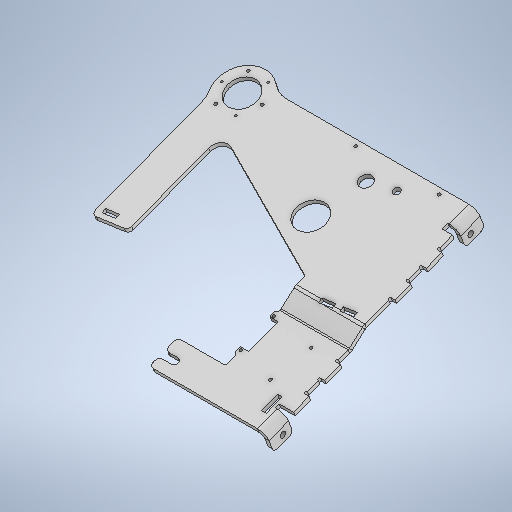
# Autodesk Inventor part: 21-30-220-B1
Saved by Autodesk Inventor 2025.2 (Build 292293000, 293)
## iProperties
Created: 2024-12-03
Part Number: 21-30-220-B1
Material: Generic
Document SubType Name: Sheet Metal
Designer: Zvonko.Gabric
Density: 1 g/cm^3
Sheet Metal Rule: Default_mm
Appearance: Default
Author: Zvonko.Gabric
Autodesk Inventor part; units mm, degrees
ref_plane "YZ Plane" through (0, 0, 0) normal (1, 0, 0) x (0, 1, 0)
ref_plane "XZ Plane" through (0, 0, 0) normal (0, 1, 0) x (-1, 0, 0)
ref_plane "XY Plane" through (0, 0, 0) normal (0, 0, 1) x (1, 0, 0)
sketch "Sketch1" plane through (0, 0, 0) normal (0, 1, 0) x (-1, 0, 0)
  line L0 (0, 0) -> (135, 0)
  line L1 (140, -5) -> (140, -6.9)
  line L2 (135, -11.9) -> (124, -11.9)
  line L3 (124, -11.9) -> (124, -20.1) construction
  line L4 (124, -20.1) -> (135, -20.1)
  line L5 (140, -25.1) -> (140, -31)
  line L6 (135, -36) -> (85, -36)
  arc A0 (124, -11.9) -> (124, -20.1) centre (124, -16) ccw
  arc A1 (140, -5) -> (135, 0) centre (135, -5) ccw
  arc A2 (135, -11.9) -> (140, -6.9) centre (135, -6.9) ccw
  arc A3 (140, -25.1) -> (135, -20.1) centre (135, -25.1) ccw
  arc A4 (135, -36) -> (140, -31) centre (135, -31) ccw
  line L7 (0, 0) -> (0, -25)
  line L8 (0, -25) -> (12.5, -25)
  line L9 (12.5, -25) -> (12.5, -30)
  line L10 (12.5, -30) -> (-5, -30)
  line L11 (-5, -30) -> (-5, -50)
  line L12 (-5, -50) -> (0, -50)
  arc A5 (0, -53) -> (0, -50) centre (0, -51.5) ccw
  arc A6 (0, -70) -> (0, -67) centre (0, -68.5) ccw
  line L13 (0, -53) -> (0, -67)
  line L14 (0, -70) -> (-5, -70)
  line L15 (-5, -70) -> (-5, -90)
  line L16 (-5, -90) -> (0, -90)
  line L17 (0, -93) -> (0, -162)
  line L18 (0, -165) -> (-5, -165)
  arc A7 (0, -93) -> (0, -90) centre (0, -91.5) ccw
  arc A8 (0, -165) -> (0, -162) centre (0, -163.5) ccw
  line L19 (-5, -165) -> (-5, -185)
  line L20 (-5, -185) -> (0, -185)
  line L21 (0, -185) -> (0, -186.5) construction
  arc A9 (0, -188) -> (0, -185) centre (0, -186.5) ccw
  line L22 (0, -186.5) -> (0, -188) construction
  line L23 (0, -188) -> (0, -202)
  line L24 (0, -195) -> (4.1858, -195) construction
  arc A10 (0, -205) -> (0, -202) centre (0, -203.5) ccw
  line L25 (0, -205) -> (-5, -205)
  line L26 (-5, -205) -> (-5, -225)
  line L27 (-5, -215) -> (-2.9961, -215) construction
  arc A11 (0, -228) -> (0, -225) centre (0, -226.5) ccw
  line L28 (0, -225) -> (-5, -225)
  line L29 (0, -228) -> (0, -243.9)
  line L30 (0, -243.9) -> (12.5, -243.9)
  line L31 (12.5, -243.9) -> (12.5, -251.27)
  line L32 (0.67, -276.27) -> (15.8838, -276.27)
  line L33 (12.5, -251.27) -> (0.67, -251.27)
  line L34 (0.67, -251.27) -> (0.67, -276.27)
  line L35 (15.8838, -276.27) -> (229.1473, -276.27)
  arc A12 (248.4086, -283.27) -> (294.835, -247.5396) centre (267.67, -260.27) ccw
  line L36 (292, -98.151) -> (292, -234.8092)
  arc A13 (292, -234.8092) -> (294.835, -247.5396) centre (322, -234.8092) ccw
  arc A14 (248.4086, -283.27) -> (229.1473, -276.27) centre (229.1473, -306.27) ccw
  line L37 (286.3907, -93.1882) -> (256.3907, -96.8718)
  line L38 (252, -101.8345) -> (252, -200.675)
  line L39 (235.0676, -211.6144) -> (83.7669, -143.3949)
  arc A15 (235.0676, -211.6144) -> (252, -200.675) centre (240, -200.675) ccw
  arc A16 (292, -98.151) -> (286.3907, -93.1882) centre (287, -98.151) ccw
  arc A17 (256.3907, -96.8718) -> (252, -101.8345) centre (257, -101.8345) ccw
  line L40 (82, -39) -> (82, -48)
  line L41 (85, -51) -> (85, -51)
  line L42 (85, -51.873) -> (85, -57)
  line L43 (84, -58) -> (76, -58)
  line L44 (75, -59) -> (75, -94.7)
  line L45 (76, -95.7) -> (84, -95.7)
  line L46 (85, -96.7) -> (85, -101.827)
  line L47 (85, -102.7) -> (85, -102.7)
  line L48 (82, -105.7) -> (82, -140.66)
  arc A18 (85, -36) -> (82, -39) centre (85, -39) ccw
  arc A19 (82, -48) -> (84.25, -50.9047) centre (85, -48) ccw
  arc A20 (84.25, -102.7953) -> (82, -105.7) centre (85, -105.7) ccw
  arc A21 (85, -51.873) -> (84.25, -50.9047) centre (84, -51.873) ccw
  arc A22 (84, -58) -> (85, -57) centre (84, -57) ccw
  arc A23 (76, -58) -> (75, -59) centre (76, -59) ccw
  arc A24 (75, -94.7) -> (76, -95.7) centre (76, -94.7) ccw
  arc A25 (85, -96.7) -> (84, -95.7) centre (84, -96.7) ccw
  arc A26 (84.25, -102.7953) -> (85, -101.827) centre (84, -101.827) ccw
  arc A27 (82, -140.66) -> (83.7669, -143.3949) centre (85, -140.66) ccw
  point P0 (140, 0)
  point P1 (140, -20.1)
  point P2 (140, -36)
  point P3 (82, -36)
  point P4 (1.5, -68.5)
  point P5 (1.5, -51.5)
  point P6 (7.9419, -276.27)
  point P7 (242.2928, -276.27)
  point P8 (292, -242.7186)
  point P9 (82, -142.5982)
  point P10 (82, -51)
  point P11 (85, -58)
  point P12 (75, -58)
  point P13 (75, -95.7)
  point P14 (85, -95.7)
  point P15 (82, -102.7)
  point P16 (140, -28.05)
  point P17 (0.67, -263.77)
  point P18 (140, -5.95)
  point P19 (271.3907, -95.03)
  dimension "d0" = 140
  dimension "d2" = 36
  dimension "d3" = 8.2
  dimension "d4" = 16
  dimension "d5" = 16
  dimension "d6" = 5
  dimension "d7" = 5
  dimension "d8" = 25
  dimension "d9" = 5
  dimension "d10" = 12.5
  dimension "d12" = 20
  dimension "d18" = 17
  dimension "d19" = 14
  dimension "d20" = 1.5
  dimension "d21" = 5
  dimension "d22" = 5
  dimension "d23" = 20
  dimension "d24" = 17
  dimension "d25" = 5
  dimension "d26" = 1.5
  dimension "d27" = 20
  dimension "d28" = 5
  dimension "d29" = 5
  dimension "d31" = 3
  dimension "d32" = 3
  dimension "d33" = 1.5
  dimension "d34" = 69
  dimension "d35" = 5
  dimension "d36" = 75
  dimension "d37" = 20
  dimension "d38" = 1.5
  dimension "d39" = 14
  dimension "d40" = 5
  dimension "d41" = 5
  dimension "d42" = 20
  dimension "d43" = 1.5
  dimension "d44" = 15.9
  dimension "d46" = 276.27
  dimension "d48" = 12.5
  dimension "d49" = 90
  dimension "d50" = 11.83
  dimension "d51" = 25
  dimension "d74" = 60
  dimension "d76" = 292
  dimension "d77" = 30
  dimension "d78" = 40
  dimension "d79" = 97
  dimension "d80" = 12
  dimension "d81" = 5
  dimension "d85" = 58
  dimension "d86" = 37.7
  dimension "d88" = 22
  dimension "d89" = 7
  dimension "d92" = 7
  dimension "d93" = 3
  dimension "d94" = 3
  dimension "d95" = 90
  dimension "d96" = 65
  dimension "d97" = 3
  dimension "d98" = 1
  dimension "d108" = 3
  dimension "d109" = 34.96
  dimension "d119" = 16
  dimension "d164" = 267
  measures "d0" distance of L0.start point (140, 0)
  measures "d2" distance between parallel lines of L6 L0
  measures "d3" distance of L2.end L3.end
  measures "d4" distance from line of L0 point (124, -16)
  measures "d5" distance between parallel lines of L1 L3
  measures "d6" radius of A1
  measures "d7" radius of A3
  measures "d8" distance of L0.start L7.end
  measures "d9" distance of L8.end L9.end
  measures "d10" distance of L7.end L8.end
  measures "d12" distance of L10.end L11.end
  measures "d18" distance of A6.centre A5.centre
  measures "d19" distance of L13.start L13.end
  measures "d20" radius of A6
  measures "d21" distance between parallel lines of L11 L13
  measures "d22" distance of L11.end L12.end
  measures "d23" distance of L14.start L12.end
  measures "d24" distance of point (1.5, -68.5) point (1.5, -51.5)
  measures "d25" distance from line of L15 A6.centre
  measures "d26" radius of A5
  measures "d27" distance of L14.end L15.end
  measures "d28" distance of L15.end L16.end
  measures "d29" distance of L18.start L18.end
  measures "d31" diameter of A7
  measures "d32" diameter of A8
  measures "d33" distance from line of L18 A8.centre
  measures "d34" distance of L17.start L17.end
  measures "d35" distance from line of L11 A5.centre
  measures "d36" distance between parallel lines of L18 L16
  measures "d37" distance of L18.end L19.end
  measures "d38" distance of L20.end L21.end
  measures "d39" distance of L22.end L23.end
  measures "d40" distance from line of L19 A10.centre
  measures "d41" distance between parallel lines of L23 L26
  measures "d42" distance of L25.end L26.end
  measures "d43" distance from line of A10.centre L25
  measures "d44" distance of L29.start L29.end
  measures "d46" distance from line of L0 point (7.942, -276.27)
  measures "d48" distance of L29.end L30.end
  measures "d49" angle of L31 L33
  measures "d50" distance of L31.end L33.end
  measures "d51" distance between parallel lines of L32 L33
  measures "d74" diameter of A12
  measures "d76" distance between parallel lines of L29 L36
  measures "d77" radius of A13
  measures "d78" distance between parallel lines of L36 L38
  measures "d79" angle of L36 L37
  measures "d80" radius of A15
  measures "d81" radius of A16
  measures "d85" distance between parallel lines of L5 L40
  measures "d86" distance of point (75, -58) point (75, -95.7)
  measures "d88" distance between parallel lines of L6 L43
  measures "d89" distance of L41.end point (85, -58)
  measures "d92" distance of point (85, -95.7) L47.start
  measures "d93" distance of point (82, -51) L41.end
  measures "d94" distance of L47.start point (82, -102.7)
  measures "d95" angle of L47 L48
  measures "d96" distance from line of point (140, -28.05) L44
  measures "d97" radius of A18
  measures "d98" radius of A21
  measures "d108" radius of A27
  measures "d109" distance of L48.start L48.end
  measures "d119" distance from line of L35 A12.centre
  measures "d164" distance from line of A12.centre L34
extrude "Plate2" add sketch "Sketch1" along normal blind 5
sketch "Sketch7" plane through (0, 5, 0) normal (0, 1, 0) x (1, 0, 0)
  line L0 (-82, 105.7) -> (-82, 140.66) projected
  line L1 (-82, 106.8) -> (0, 106.8)
  line L2 (0, 93) -> (0, 162) projected
  line L3 (0, 0) -> (-135, 0) projected
  point P0 (-82, 131.7303)
  dimension "d100" = 106.8
  constraints: 2 end point, 2 point on line, 1 horizontal
  measures "d100" distance between parallel lines of L3 L1
fold "Fold3" angle 20.9 bend radius 5 thickness 5 k factor 0.44 line from (-82, 5, -106.8) to (0, 5, -106.8) line at bend centre moving side (0, 0, -1) folds toward (0, 1, 0)
sketch "Sketch9" plane through (-229.1473, 60.6459, -266.147) normal (0, -0.9342045, -0.356738) x (1, 0, 0)
  line L0 (147.1473, 168.1568) -> (147.1473, 135.61) projected
  line L1 (147.1473, 146.0404) -> (229.1473, 146.0404)
  line L2 (229.1473, 114.27) -> (229.1473, 168.1568) projected
  line L3 (94.1473, 270.2704) -> (229.1473, 270.2704) projected
  dimension "d110" = 124.23
  constraints: 2 end point, 2 point on line, 1 horizontal
  measures "d110" distance between parallel lines of L3 L1
fold "Fold4" angle 20.9 bend radius 5 thickness 5 k factor 0.44 line from (-82, 8.5477, -129.7154) to (0, 8.5477, -129.7154) line at bend centre moving side (0, -0.356738, 0.9342045) folds toward (0, -0.9342045, -0.356738)
sketch "Sketch10" plane through (-229.1473, 65.3169, -264.3634) normal (0, 0.9342045, 0.356738) x (1, 0, 0)
  circle A0 centre (-38.5227, -16) radius 17.5
  line L0 (228.4773, 0) -> (228.4773, -25) projected
  line L1 (0, 0) -> (228.4773, 0) projected
  point P0 (229.1473, -270.2704)
  point P1 (228.4773, -12.5)
  dimension "d121" = 267
  dimension "d122" = 16
  dimension "d123" = 35
  constraints: 1 centre point, 1 midpoint
  measures "d121" horizontal distance of A0.centre point (228.477, -12.5)
  measures "d122" distance from line of L1 A0.centre
  measures "d123" diameter of A0
extrude "Extrusion1" cut sketch "Sketch10" against normal blind 10
sketch "Sketch11" plane through (-229.1473, 65.3169, -264.3634) normal (0, 0.9342045, 0.356738) x (1, 0, 0)
  line L0 (-64.6699, -16) -> (-19.5412, -16) construction
  circle A0 centre (-38.5227, -16) radius 17.5 projected
  line L1 (-38.5227, -33.5) -> (-38.5227, 1.5) construction
  circle A1 centre (-62.5227, -16) radius 1.25
  circle A2 centre (-38.5227, -16) radius 24 construction
  circle A3 centre (-38.5227, -16) radius 24 construction
  circle A4 centre (-26.5227, -36.7846) radius 1.25
  circle A5 centre (-38.5227, -16) radius 24 construction
  circle A6 centre (-26.5227, 4.7846) radius 1.25
  point P0 (229.1473, -270.2704)
  dimension "d127" = 48
  dimension "d126" = 2.5
  dimension "d130" = 360
  constraints: 4 end point, 3 centre point, 3 coincident, 2 point on circle, 1 horizontal, 1 horizontal alignment, 1 point on line, 19 other
  measures "d126" diameter of A1
extrude "Extrusion2" cut sketch "Sketch11" against normal blind 10 contours A1 | A4 | A6
sketch "Sketch12" plane through (-229.1473, 65.3169, -264.3634) normal (0, 0.9342045, 0.356738) x (1, 0, 0)
  circle A0 centre (-38.5227, -16) radius 17.5 projected
  circle A1 centre (-26.5227, -36.7846) radius 1.25 projected
  circle A2 centre (-38.5227, -16) radius 24 construction
  circle A3 centre (-50.5227, -36.7846) radius 1.75
  line L0 (-50.5227, -36.7846) -> (-38.5227, -16) construction
  line L1 (-62.5227, -16) -> (-38.5227, -16) construction
  line L2 (-26.5227, -36.7846) -> (-38.5227, -16) construction
  circle A4 centre (-14.5227, -16) radius 1.75
  line L3 (-26.5227, 4.7846) -> (-38.5227, -16) construction
  circle A5 centre (-50.5227, 4.7846) radius 1.75
  line L4 (-38.5227, -16) -> (-50.5227, 4.7846) construction
  point P0 (229.1473, -270.2704)
  dimension "d134" = 3.5
  dimension "d135" = 60
  dimension "d138" = 360
  dimension "d140" = 120
  constraints: 10 end point, 4 centre point, 3 point on circle, 1 coincident, 1 horizontal, 16 other
  measures "d134" diameter of A3
  measures "d135" angle of L0 L1
  measures "d140" angle of L0 L4
extrude "Extrusion3" cut sketch "Sketch12" against normal blind 10 contours A3 | A4 | A5
thread "Thread1" size "M3x0.5" class "6H" standard "ANSI Metric M Profile" length 20
thread "Thread2" size "M3x0.5" class "6H" standard "ANSI Metric M Profile" length 20
thread "Thread3" size "M3x0.5" class "6H" standard "ANSI Metric M Profile" length 20
thread "Thread4" size "M4x0.7" class "6H" standard "ISO Metric profile" length 5
thread "Thread5" size "M4x0.7" class "6H" standard "ANSI Metric M Profile" length 5
thread "Thread6" size "M4x0.7" class "6H" standard "ISO Metric profile" length 5
sketch "Sketch13" plane through (-229.1473, 65.3169, -264.3634) normal (0, 0.9342045, 0.356738) x (1, 0, 0)
  circle A0 centre (106.4773, -83) radius 17.5
  line L0 (0, 0) -> (228.4773, 0) projected
  line L1 (228.4773, 0) -> (228.4773, -25) projected
  point P0 (229.1473, -270.2704)
  dimension "d155" = 83
  dimension "d156" = 122
  dimension "d157" = 35
  constraints: 1 centre point
  measures "d155" distance from line of L0 A0.centre
  measures "d156" distance from line of L1 A0.centre
  measures "d157" diameter of A0
extrude "Extrusion4" cut sketch "Sketch13" against normal blind 10
sketch "Sketch14" plane through (-229.1473, 65.3169, -264.3634) normal (0, 0.9342045, 0.356738) x (1, 0, 0)
  circle A0 centre (122.4773, -29.5) radius 7.5
  line L0 (228.4773, 0) -> (228.4773, -25) projected
  line L1 (0, 0) -> (228.4773, 0) projected
  circle A1 centre (153.4773, -23) radius 4
  circle A2 centre (188.4773, -6) radius 1.75
  circle A3 centre (88.4773, -6) radius 1.75
  point P0 (229.1473, -270.2704)
  point P1 (228.4773, -12.5)
  dimension "d172" = 15
  dimension "d173" = 106
  dimension "d174" = 29.5
  dimension "d175" = 75
  dimension "d176" = 23
  dimension "d177" = 8
  dimension "d178" = 40
  dimension "d179" = 6
  dimension "d180" = 3.5
  dimension "d181" = 140
  dimension "d182" = 6
  dimension "d183" = 3.5
  constraints: 4 centre point, 1 midpoint
  measures "d172" diameter of A0
  measures "d173" horizontal distance of point (228.477, -12.5) A0.centre
  measures "d174" distance from line of L1 A0.centre
  measures "d175" distance from line of L0 A1.centre
  measures "d176" distance from line of L1 A1.centre
  measures "d177" diameter of A1
  measures "d178" distance from line of L0 A2.centre
  measures "d179" distance from line of L1 A2.centre
  measures "d180" diameter of A3
  measures "d181" distance from line of L0 A3.centre
  measures "d182" distance from line of L1 A3.centre
  measures "d183" diameter of A2
extrude "Extrusion5" cut sketch "Sketch14" against normal blind 10
thread "Thread7" size "M4x0.7" class "6H" standard "ISO Metric profile" length 5
thread "Thread8" size "M4x0.7" class "6H" standard "ISO Metric profile" length 5
sketch "Sketch15" plane through (-135, -40.6409, -10.4571) normal (0, 0.9342045, 0.356738) x (1, 0, 0)
  circle A0 centre (53, 55.5) radius 1.65
  circle A1 centre (53, 98.2) radius 1.65
  line L0 (60, 59) -> (60, 94.7) projected
  line L1 (51, 58) -> (59, 58) projected
  circle A2 centre (98, 45.5) radius 1.65
  line L2 (135, 25) -> (135, 0) projected
  line L3 (135, 0) -> (0, 0) projected
  circle A3 centre (105, 90) radius 1.65
  line L4 (114.5, 37) -> (120, 37)
  line L5 (120, 37) -> (120, 16.5)
  line L6 (120, 16.5) -> (114.5, 16.5)
  line L7 (114.5, 16.5) -> (114.5, 37)
  line L8 (114.5, 37) -> (120, 16.5) construction
  line L9 (120, 37) -> (114.5, 16.5) construction
  point P0 (135, 4.7291)
  point P1 (117.25, 26.75)
  dimension "d190" = 3.3
  dimension "d191" = 7
  dimension "d192" = 7
  dimension "d193" = 42.7
  dimension "d194" = 2.5
  dimension "d195" = 3.3
  dimension "d196" = 37
  dimension "d197" = 45.5
  dimension "d198" = 3.3
  dimension "d199" = 3.3
  dimension "d200" = 90
  dimension "d201" = 30
  dimension "d202" = 20.5
  dimension "d203" = 15
  dimension "d204" = 20.5
  dimension "d205" = 16.5
  constraints: 12 end point, 4 centre point, 2 midpoint, 2 parallel, 1 horizontal, 1 perpendicular
  measures "d190" diameter of A0
  measures "d191" distance from line of A0.centre L0
  measures "d192" distance from line of L0 A1.centre
  measures "d193" distance of A1.centre A0.centre
  measures "d194" distance from line of L1 A0.centre
  measures "d195" diameter of A1
  measures "d196" distance from line of L2 A2.centre
  measures "d197" distance from line of L3 A2.centre
  measures "d198" diameter of A2
  measures "d199" diameter of A3
  measures "d200" distance from line of L3 A3.centre
  measures "d201" distance from line of L2 A3.centre
  measures "d202" distance of L6.end L4.start
  measures "d203" distance between parallel lines of L2 L5
  measures "d204" distance between parallel lines of L2 L7
  measures "d205" distance between parallel lines of L3 L6
extrude "Extrusion6" cut sketch "Sketch15" against normal blind 10
thread "Thread9" size "M4x0.7" class "6H" standard "ISO Metric profile" length 5
thread "Thread10" size "M4x0.7" class "6H" standard "ISO Metric profile" length 5
thread "Thread11" size "M4x0.7" class "6H" standard "ISO Metric profile" length 5
thread "Thread12" size "M4x0.7" class "6H" standard "ISO Metric profile" length 5
sketch "Sketch16" plane through (0, -41.0645, -37.3795) normal (-1, 0, 0) x (0, -1, 0)
  line L0 (-0.4236, 26.9225) -> (-9.342, 3.5674)
  line L1 (-9.342, 3.5674) -> (14.9473, -5.7078)
  line L2 (14.9473, -5.7078) -> (23.8657, 17.6473)
  line L3 (23.8657, 17.6473) -> (-0.4236, 26.9225)
  constraints: 8 end point
edge flange "Flange1" height 26 angle 90 thickness 5 bend radius 5 thickness toward (-1, 0, 0) relief tear relief width 5 relief depth 2.5 edges at (0, -36.1817, -22.1346) wall of the first edge with corners at (0, -40.6409, -10.4571) (0, -31.7224, -33.8122) (0, -56.0118, -43.0874) (0, -64.9302, -19.7322)
bend "Bend1"
corner "Corner1"
fillet "Fillet1" radius 5 1 edges at (-2.5, -64.9302, -19.7322)
fillet "Fillet2" radius 5 1 edges at (-2.5, -56.0118, -43.0874)
sketch "Sketch18" plane through (-0.67, 47.0564, -244.5756) normal (-1, 0, 0) x (0, -1, 0)
  line L0 (-13.5895, -21.5714) -> (-4.671, 1.7837)
  line L1 (-4.671, 1.7837) -> (14.9473, -5.7078)
  line L2 (14.9473, -5.7078) -> (6.0288, -29.0629)
  line L3 (6.0288, -29.0629) -> (-13.5895, -21.5714)
  constraints: 8 end point
edge flange "Flange2" height 26 angle 90 thickness 5 bend radius 5 thickness toward (-1, 0, 0) relief tear relief width 5 relief depth 2.5 edges at (-0.67, 56.1867, -254.4695) wall of the first edge with corners at (-0.67, 60.6459, -266.147) (-0.67, 51.7274, -242.7919) (-0.67, 32.1091, -250.2834) (-0.67, 41.0276, -273.6385)
bend "Bend2"
corner "Corner2"
fillet "Fillet3" radius 5 2 edges at (-3.17, 41.0276, -273.6385) (-3.17, 32.1091, -250.2834)
sketch "Sketch19" plane through (-5, -41.0645, -37.3795) normal (-1, 0, 0) x (0, -0.356738, 0.9342045)
  circle A0 centre (10, -7.85) radius 3.4
  line L0 (20, -16) -> (5, -16) projected
  line L1 (25, 0) -> (25, -11) projected
  point P0 (20.2709, 51.6973)
  dimension "d239" = 8.15
  dimension "d240" = 15
  dimension "d241" = 6.8
  constraints: 1 centre point
  measures "d239" distance from line of L0 A0.centre
  measures "d240" distance from line of L1 A0.centre
  measures "d241" diameter of A0
sketch "Sketch20" plane through (-5.67, 55.9749, -267.9307) normal (-1, 0, 0) x (0, -0.356738, 0.9342045)
  circle A0 centre (15, -7.75) radius 3.4
  line L0 (0, 0) -> (0, -11) projected
  line L1 (5, -16) -> (20, -16) projected
  point P0 (270.2704, 43.2891)
  dimension "d242" = 15
  dimension "d243" = 8.25
  dimension "d244" = 6.8
  constraints: 1 centre point
  measures "d242" distance from line of L0 A0.centre
  measures "d243" distance from line of L1 A0.centre
  measures "d244" diameter of A0
extrude "Extrusion8" cut sketch "Sketch20" against normal blind 15
extrude "Extrusion9" cut sketch "Sketch19" against normal blind 10
thread "Thread13" size "M8x1.25" class "6H" standard "ISO Metric profile" length 5
thread "Thread14" size "M8x1.25" class "6H" standard "ISO Metric profile" length 5
sketch "Sketch21" plane through (-12.5, 53.7693, -234.1232) normal (0, 0.9342045, 0.356738) x (1, 0, 0)
  line L0 (-266.2387, -141.561) -> (-2.1735, -109.1379) construction
  line L1 (-279.5, -145.749) -> (-279.5, -9.0908) projected
  line L2 (-243.8907, -147.0282) -> (-273.8907, -150.7118) projected
  line L3 (-272.3785, -144.884) -> (-257.4903, -143.056)
  line L4 (-257.4903, -143.056) -> (-258.1118, -137.994)
  line L5 (-258.1118, -137.994) -> (-273, -139.8221)
  line L6 (-273, -139.8221) -> (-272.3785, -144.884)
  line L7 (-24.5943, -114.46) -> (-25.2158, -109.398)
  line L8 (-25.2158, -109.398) -> (-40.104, -111.226)
  line L9 (-39.4825, -116.288) -> (-24.5943, -114.46)
  line L10 (-40.104, -111.226) -> (-39.4825, -116.288)
  line L11 (-39.4825, -116.288) -> (-25.2158, -109.398) construction
  line L12 (-40.104, -111.226) -> (-24.5943, -114.46) construction
  line L13 (-1.4541, -111.6187) -> (-2.0756, -106.5567)
  line L14 (-2.0756, -106.5567) -> (-16.9638, -108.3848)
  line L15 (-16.3423, -113.4467) -> (-1.4541, -111.6187)
  line L16 (-16.9638, -108.3848) -> (-16.3423, -113.4467)
  line L17 (-16.9638, -108.3848) -> (-1.4541, -111.6187) construction
  line L18 (-16.3423, -113.4467) -> (-2.0756, -106.5567) construction
  point P0 (12.5, -237.9004)
  point P1 (-272.6892, -142.353)
  point P2 (-39.7932, -113.757)
  point P3 (-32.3491, -112.843)
  point P4 (-9.2089, -110.0017)
  point P5 (-32.3491, -112.843)
  dimension "d255" = 97
  dimension "d256" = 8.15
  dimension "d259" = 97
  dimension "d261" = 5.1
  dimension "d262" = 0
  dimension "d263" = 6.5
  dimension "d264" = 15
  dimension "d267" = 234.645
  dimension "d274" = 235.646
  dimension "d279" = 5.1
  dimension "d280" = 2.55
  dimension "d281" = 23.314
  constraints: 34 end point, 4 midpoint, 3 perpendicular, 10 other
  measures "d255" angle of L1 L0
  measures "d256" distance from line of L2 L0.start
  measures "d259" angle of L1 L5
  measures "d261" distance of L5.end L3.start
  measures "d262" distance from line of L0 point (-272.689, -142.353)
  measures "d263" distance from line of L1 L5.end
  measures "d264" distance of L4.end L5.end
  measures "d267" distance of L3.end L7.start
  measures "d274" distance of point (-32.349, -112.843) L0.start
  measures "d279" distance of L14.end L16.end
  measures "d280" distance between parallel lines of L14 L0
  measures "d281" distance of point (-9.209, -110.002) point (-32.349, -112.843)
extrude "Extrusion10" cut sketch "Sketch21" against normal blind 10 contours L9 L10 L8 L7
extrude "Extrusion11" cut sketch "Sketch21" against normal blind 10 contours L15 L16 L14 L13
extrude "Extrusion12" cut sketch "Sketch21" against normal blind 10 contours L6 L5 L4 L3
equation "\"d53\" = Thickness"
equation "\"BendRadius\" = Thickness"
equation "\"BendReliefWidth\" = Thickness"
equation "\"BendReliefDepth\" = 0.5 * Thickness"
equation "\"TransitionRadius\" = BendRadius"
equation "\"JacobiRadiusSize\" = BendRadius"
equation "\"GapSize\" = Thickness"
equation "\"Thickness\" = 5"
body "Solid2"
